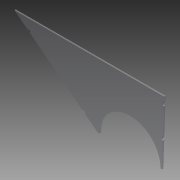
# Autodesk Inventor part: Funneling2
Saved by Autodesk Inventor 2013 (Build 170138000, 138)
## iProperties
Created: 2013-01-26
Part Number: Funneling2
Material: Polycarbonate, Clear
Document SubType Name: Modeling
Designer: actoennies
Mass: 641.602 g
Surface Area: 2385.19 cm^2
Volume: 717.676 cm^3
Density: 0.894 g/cm^3
Author: actoennies
Autodesk Inventor part; units mm, degrees
ref_plane "YZ Plane" through (0, 0, 0) normal (1, 0, 0) x (0, 1, 0)
ref_plane "XZ Plane" through (0, 0, 0) normal (0, 1, 0) x (-1, 0, 0)
ref_plane "XY Plane" through (0, 0, 0) normal (0, 0, 1) x (1, 0, 0)
sketch "Sketch1" plane through (0, 0, 0) normal (0, 0, 1) x (1, 0, 0)
  line L0 (35.56, 293.2939) -> (25.4, 0)
  line L1 (35.56, 293.2939) -> (-650.24, 293.2939)
  line L2 (-650.24, 293.2939) -> (-270.7381, 0)
  arc A0 (19.0462, 0) -> (-260.3538, 0) centre (-120.6538, 0) ccw
  line L3 (-270.7381, 0) -> (-260.3538, 0)
  line L4 (19.0462, 0) -> (25.4, 0)
  point P0 (0, 0)
  dimension "d2" = 293.2939
  dimension "d3" = 35.56
  dimension "d4" = 25.4
  dimension "d5" = 685.8
  dimension "d8" = 279.4
  dimension "d11" = 6.35
  dimension "d12" = 6.35
  constraints: 10 end point, 2 parallel, 2 point on circle, 1 centre point, 1 horizontal
  measures "d2" vertical distance of L0.start point (0, 0)
  measures "d3" horizontal distance of point (0, 0) L0.start
  measures "d4" distance of point (0, 0) L0.end
  measures "d5" distance of L0.start L1.end
  measures "d8" diameter of A0
  measures "d11" distance from line of L3.end L2
  measures "d12" distance from line of L4.start L0
extrude "Extrusion1" add sketch "Sketch1" along normal blind 6.35
sketch "Sketch2" plane through (0, 0, 6.35) normal (0, 0, 1) x (1, 0, 0)
  line L0 (25.4, 0) -> (35.56, 293.2939) projected
  line L1 (28.3345, 268.129) -> (34.6806, 267.9092)
  line L2 (27.8948, 255.4366) -> (34.241, 255.2168)
  line L3 (23.498, 128.5127) -> (29.8442, 128.2929)
  line L4 (23.0583, 115.8204) -> (29.4045, 115.6005)
  line L5 (23.0583, 115.8204) -> (23.498, 128.5127)
  line L6 (27.8948, 255.4366) -> (28.3345, 268.129)
  point P0 (0, 0)
  dimension "d21" = 12.7
  dimension "d23" = 12.7
  dimension "d24" = 25.4
  dimension "d25" = 127
  constraints: 12 end point, 5 parallel, 4 point on line, 1 perpendicular
  measures "d21" distance between parallel lines of L4 L3
  measures "d23" distance between parallel lines of L1 L2
  measures "d24" distance from line of L0.end L1
  measures "d25" distance between parallel lines of L3 L2
extrude "Extrusion2" cut sketch "Sketch2" against normal blind 6.35
sketch "Sketch3" plane through (0, 0, 6.35) normal (0, 0, 1) x (1, 0, 0)
  line L0 (-650.24, 293.2939) -> (-270.7381, 0) projected
  line L1 (-589.9473, 246.6974) -> (-586.0643, 251.7218)
  line L2 (-576.0155, 243.9557) -> (-579.8986, 238.9313)
  line L3 (-334.8449, 57.5696) -> (-338.7279, 52.5452)
  line L4 (-324.7961, 49.8035) -> (-328.6792, 44.7792)
  line L5 (-586.0643, 251.7218) -> (-576.0155, 243.9557)
  line L6 (-334.8449, 57.5696) -> (-324.7961, 49.8035)
  point P0 (0, 0)
  dimension "d28" = 6.35
  dimension "d29" = 12.7
  dimension "d30" = 12.7
  dimension "d31" = 76.2
  dimension "d32" = 304.8
  constraints: 12 end point, 4 parallel, 4 point on line, 3 perpendicular
  measures "d28" distance of L1.start L1.end
  measures "d29" distance between parallel lines of L2 L1
  measures "d30" distance between parallel lines of L3 L4
  measures "d31" distance from line of L0.start L1
  measures "d32" distance between parallel lines of L3 L2
extrude "Extrusion3" cut sketch "Sketch3" against normal blind 6.35
body "Solid1"
